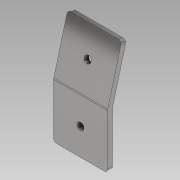
# Autodesk Inventor part: am-2847
Saved by Autodesk Inventor 2020.1 (Build 241239000, 239)
## iProperties
Category: FIRSTChoice
Company: Autodesk Inc.
Created: 2019-11-26
Part Number: am-2847
Material: Steel
Document SubType Name: Modeling
Designer: Autodesk Inc.
Density: 7.85 g/cm^3
Appearance: Steel - Polished
Catalog Web Link: https://www.andymark.com/products/15-degree-bolt-bracket
Vendor: AndyMark Inc.
Author: Autodesk Inc.
Autodesk Inventor part; units mm, degrees
ref_plane "YZ Plane" through (0, 0, 0) normal (1, 0, 0) x (0, 1, 0)
ref_plane "XZ Plane" through (0, 0, 0) normal (0, 1, 0) x (-1, 0, 0)
ref_plane "XY Plane" through (0, 0, 0) normal (0, 0, 1) x (1, 0, 0)
sketch "Sketch4" plane through (0, 0, 0) normal (0, 0, 1) x (1, 0, 0)
  line L0 (0, 0) -> (2.286, 0)
  line L1 (2.286, 0) -> (2.286, -25.4)
  line L2 (2.286, -25.4) -> (0, -25.4)
  line L3 (0, -25.4) -> (0, 0)
  line L4 (2.286, 0) -> (27.686, 0) construction
  line L5 (0.0779, 0.5917) -> (2.286, 0)
  arc A0 (0.0779, 0.5917) -> (0, 0) centre (2.286, 0) ccw
  line L6 (2.286, 0) -> (8.86, 24.5345)
  line L7 (2.286, 0) -> (27.686, 0) construction
  line L8 (8.86, 24.5345) -> (6.6519, 25.1262)
  line L9 (6.6519, 25.1262) -> (0.0779, 0.5917)
  dimension "d14" = 2.286
  dimension "d15" = 25.4
  dimension "d20" = 25.4
  dimension "d21" = 75
  dimension "d22" = 2.286
  dimension "d23" = 90
  constraints: 20 end point, 3 horizontal, 3 perpendicular, 2 parallel, 2 point on circle, 1 centre point, 1 coincident, 1 equal length
  measures "d14" distance of L1.end L2.end
  measures "d15" distance of L0.end L1.end
  measures "d20" distance of L6.start L6.end
  measures "d21" angle of L7 L6
  measures "d22" distance of L6.end L8.end
  measures "d23" angle of L8 L6
extrude "Extrusion2" add sketch "Sketch4" against normal blind 25.4
sketch "Sketch5" plane through (6.6519, 25.1262, -25.4) normal (-0.9659258, 0.258819, 0) x (0, 0, 1)
  line L0 (25.4, 0) -> (0, 0) projected
  line L1 (25.4, -25.4) -> (0, -25.4) projected
  point P0 (25.4, -25.9917)
  point P1 (12.7, -12.7)
  point P2 (12.7, 0)
  dimension "d26" = 12.7
  constraints: 1 midpoint, 1 vertical alignment
  measures "d26" distance from line of point (12.7, -12.7) L1
sketch "Sketch6" plane through (0, -25.4, 0) normal (-1, 0, 0) x (0, 0, 1)
  line L0 (0, 0) -> (-25.4, 0) projected
  line L1 (0, 25.4) -> (-25.4, 25.4) projected
  point P0 (-12.7, 12.7)
  point P1 (-12.7, 0)
  dimension "d27" = 12.7
  constraints: 1 midpoint, 1 vertical alignment
  measures "d27" distance from line of L1 point (-12.7, 12.7)
hole "Hole2" at (3.3649, 12.8589, -12.7) direction (0.9659258, -0.258819, 0) diameter 3.2512 end through all
hole "Hole3" at (0, -12.7, -12.7) direction (1, 0, 0) diameter 3.2512 end through all
fillet "Fillet2" radius 1.524 4 edges at (7.756, 24.8303, 0) (7.756, 24.8303, -25.4) (1.143, -25.4, -25.4) (1.143, -25.4, 0)
body "Solid2"
